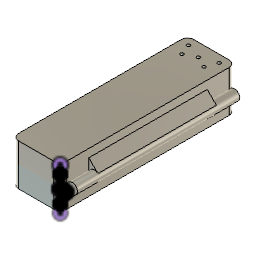
toothbrush box (Autodesk Fusion 360 design; units mm, degrees)
part number: 2025-10-09-22-59-32-254
Autodesk Fusion 360 part; units mm, degrees
sketch "Sketch1" plane through (0, 0, 0) normal (0, 0, 1) x (1, 0, 0)
  line L0 (6, 0) -> (38, 0)
  line L1 (44, -6) -> (44, -154)
  line L2 (38, -160) -> (6, -160)
  line L3 (0, -154) -> (0, -6)
  arc A0 (6, 0) -> (0, -6) centre (6, -6) ccw
  arc A1 (44, -6) -> (38, 0) centre (38, -6) ccw
  arc A2 (0, -154) -> (6, -160) centre (6, -154) ccw
  arc A3 (38, -160) -> (44, -154) centre (38, -154) ccw
  point P0 (0, -160)
  dimension "d1" = 160
  dimension "d2" = 44
  dimension "d3" = 6
  dimension "d4" = 6
  dimension "d5" = 6
  dimension "d6" = 6
  constraint horizontal L0
  constraint vertical L1
  constraint horizontal L2
  constraint vertical L3
  constraint coincident origin L0
  constraint coincident origin L3
  constraint tangent L0 A0
  constraint tangent L3 A0
  constraint tangent L0 A1
  constraint tangent L1 A1
  constraint coincident P0 L3
  constraint coincident P0 L2
  constraint tangent L3 A2
  constraint tangent L2 A2
  constraint tangent L2 A3
  constraint tangent L1 A3
  measures "d1" distance of origin P0
  measures "d2" distance of origin L1
  measures "d3" radius of A0
  measures "d4" radius of A1
  measures "d5" radius of A2
  measures "d6" radius of A3
extrude "Extrude1" add sketch "Sketch1" along normal blind 19 makes body 1
shell "Shell1" thickness 2 removed faces 1 at (14.6667, -55.3333, 19) on bodies 1
sketch "Sketch3" plane through (0, 0, 2) normal (0, 0, 1) x (-1, 0, 0)
  arc A0 (-2, 154) -> (-6, 158) centre (-6, 154) ccw
  line L0 (-6, 158) -> (-38, 158)
  arc A1 (-38, 158) -> (-42, 154) centre (-38, 154) ccw
  line L1 (-42, 154) -> (-42, 6)
  arc A2 (-42, 6) -> (-38, 2) centre (-38, 6) ccw
  line L2 (-38, 2) -> (-6, 2)
  arc A3 (-6, 2) -> (-2, 6) centre (-6, 6) ccw
  line L3 (-2, 6) -> (-2, 154)
  line L4 (-22, 2) -> (-22, 22) construction
  line L5 (-2, 22) -> (-42, 22)
  line L6 (-42, 22) -> (-42, 25)
  line L7 (-42, 25) -> (-2, 25)
  line L8 (-2, 25) -> (-2, 22)
  dimension "d10" = 20
  dimension "d11" = 3
  constraint midpoint L2 L4.start
  constraint perpendicular L2 L4
  constraint horizontal L5
  constraint vertical L6
  constraint horizontal L7
  constraint vertical L8
  constraint coincident L3 L5.start
  measures "d10" distance of L4.start L4.end
  measures "d11" distance of L5.start L7.end
extrude "Extrude2" add sketch "Sketch3" along normal blind 2 contours L1 L3 L5 L6 L7 L8 bodies 1
copy_body "CopyPasteBodies1" bodies 1 makes body 2
move_body "Move1" bodies 2 to x (1, 0, 0) y (0, 1, 0) z (0, 0, 1) at (0, 0, 20)
extrude "Extrude3" cut 1 faces at (28.6667, -23, 24) along direction (0, 0, -1) blind 2 on bodies 2 bodies 2
sketch "Sketch4" plane through (0, 0, 22) normal (0, 0, 1) x (-1, 0, 0)
  line L0 (-42, 154) -> (-42, 6)
  arc A0 (-42, 6) -> (-38, 2) centre (-38, 6) ccw
  line L1 (-38, 2) -> (-6, 2)
  arc A1 (-6, 2) -> (-2, 6) centre (-6, 6) ccw
  line L2 (-2, 6) -> (-2, 154)
  arc A2 (-2, 154) -> (-6, 158) centre (-6, 154) ccw
  line L3 (-6, 158) -> (-38, 158)
  arc A3 (-38, 158) -> (-42, 154) centre (-38, 154) ccw
  line L4 (-22, 2) -> (-22, 22) construction
  circle A4 centre (-8, 7) radius 1.5
  circle A5 centre (-22, 12) radius 1.5
  circle A6 centre (-12, 17) radius 1.5
  circle A7 centre (-36, 7) radius 1.5
  circle A8 centre (-12, 17) radius 1.5
  line L5 (-32, 17) -> (-31, 17)
  circle A9 centre (-32, 17) radius 1.5
  dimension "d17" = 20
  dimension "d18" = 3
  dimension "d19" = 3
  dimension "d20" = 3
  dimension "d22" = 3
  dimension "d23" = 3
  dimension "d24" = 3
  constraint midpoint L1 L4.start
  constraint perpendicular L1 L4
  constraint midpoint L4 A5.centre
  constraint perpendicular L4 L5
  constraint coincident L5.start A9.centre
  measures "d17" distance of L4.start L4.end
  measures "d18" diameter of A4
  measures "d19" diameter of A5
  measures "d20" diameter of A6
  measures "d22" diameter of A7
  measures "d23" diameter of A8
  measures "d24" diameter of A9
extrude "Extrude4" cut sketch "Sketch4" against normal blind 40 contours A4 | A5 | A6 A8 | A7 | A9 bodies 1 2
move_body "Move2" bodies 2 to x (-1, 0, 0) y (0, 1, 0) z (0, 0, -1) at (84, 0, 44)
move_body "Move3" bodies 2 to x (1, 0, 0) y (0, 1, 0) z (0, 0, 1) at (-40, 0, 14)
sketch "Sketch6" plane through (0, -160, 0) normal (0, -1, 0) x (1, 0, 0)
  line L0 (6, 0) -> (38, 0)
  line L1 (38, 0) -> (38, 19)
  line L2 (38, 19) -> (6, 19)
  line L3 (6, 19) -> (6, 0)
  line L4 (44, 19) -> (53.7, 19) construction
  circle A0 centre (49, 19) radius 1.5
  circle A1 centre (49, 19) radius 1.7
  circle A2 centre (49, 19) radius 4.7
  line L5 (44, 19) -> (44.3, 19)
  line L6 (52.3234, 15.6766) -> (44, 7.3532)
  line L7 (52.3234, 22.3234) -> (44, 30.6468)
  line L8 (44, 38) -> (44, 19)
  line L9 (44, 19) -> (44, 38)
  line L10 (44, 0) -> (44, 19)
  line L11 (44, 19) -> (44, 0)
  dimension "d28" = 3
  dimension "d29" = 0.2
  dimension "d30" = 3
  dimension "d31" = 5
  dimension "d32" = 45
  constraint horizontal L4
  constraint coincident L4 A0.centre
  constraint concentric A0 A1
  constraint concentric A0 A2
  constraint coincident L4 L5.end
  constraint coincident A2 L5.end
  constraint coincident A2 L6.start
  constraint coincident A2 L7.start
  constraint perpendicular L6 L7
  constraint coincident L7.end L8
  constraint coincident L6.end L11
  constraint coincident L4.start L5.start
  constraint tangent A2 L7
  constraint tangent A2 L6
  constraint coincident L4.end A2
  measures "d28" diameter of A0
  measures "d29" distance of A0 A1
  measures "d30" distance of A1 A2
  measures "d31" distance of L4.start A0.centre
  measures "d32" angle of L6 L10
ref_plane "WorkPlane2" through (2, -154, 2) normal (0, -1, 0) x (1, 0, 0)
extrude "Extrude5" add sketch "Sketch6" against normal blind 12 from surface at -6 contours A0 | A1 | A2 | A2 L5 L6 L10 L11 bodies 1
ref_plane "WorkPlane3" through (2, -6, 2) normal (0, -1, 0) x (1, 0, 0)
extrude "Extrude6" add 1 faces at (46.8745, -142, 14.0099) along direction (0, 1, 0) blind 8 on bodies 1 bodies 1
extrude "Extrude7" add sketch "Sketch6" along normal blind 20 from surface at -154 contours A0 | A1 | A2 | A2 L5 L6 L10 L11 bodies 1
extrude "Extrude8" add sketch "Sketch6" against normal up to surface (148 mm away) from surface at -6 contours A0 bodies 1
extrude "Extrude9" add sketch "Sketch6" against normal blind 108 from surface at -26 contours A2 | A2 L5 L7 L8 L9 bodies 1 2
